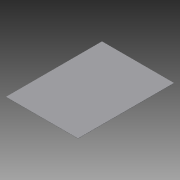
# Autodesk Inventor part: Sol
Saved by Autodesk Inventor 2015 SP1 (Build 190203100, 203)
## iProperties
Created: 2015-04-25
Part Number: Sol
Material: Générique
Document SubType Name: Modeling
Designer: Cyril
Density: 1 g/cm^3
Appearance: Par défaut
Author: Cyril
Autodesk Inventor part; units mm, degrees
ref_plane "YZ Plane" through (0, 0, 0) normal (1, 0, 0) x (0, 1, 0)
ref_plane "XZ Plane" through (0, 0, 0) normal (0, 1, 0) x (-1, 0, 0)
ref_plane "XY Plane" through (0, 0, 0) normal (0, 0, 1) x (1, 0, 0)
sketch "Sketch1" plane through (0, 0, 0) normal (0, 0, 1) x (1, 0, 0)
  line L0 (1500, 2000) -> (-1500, 2000)
  line L1 (-1500, 2000) -> (-1500, -2000)
  line L2 (-1500, -2000) -> (1500, -2000)
  line L3 (1500, -2000) -> (1500, 2000)
  line L4 (1500, 2000) -> (-1500, -2000) construction
  line L5 (-1500, 2000) -> (1500, -2000) construction
  point P0 (0, 0)
  point P1 (0, 0)
  dimension "d0" = 3000
  dimension "d1" = 4000
  constraints: 12 end point, 2 midpoint, 2 parallel, 1 coincident, 1 horizontal, 1 perpendicular
  measures "d0" distance of L0.start L0.end
  measures "d1" distance of L2.end L0.start
extrude "Extrusion1" add sketch "Sketch1" along normal blind 10
body "Solid1"
